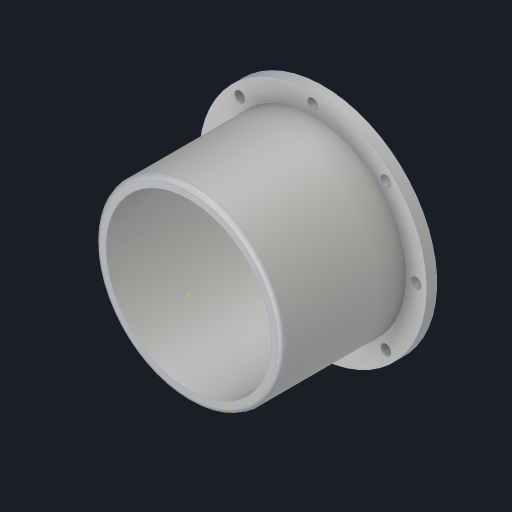
# Autodesk Inventor part: base
Saved by Autodesk Inventor 2023.4 (Build 274418000, 418)
## iProperties
Created: 2020-06-03
Part Number: base
Material: Aluminum 6061
Document SubType Name: Modeling
Designer: lenovo
Density: 2.7 g/cm^3
Appearance: Aluminum - Flat
Author: lenovo
Autodesk Inventor part; units mm, degrees
ref_plane "YZ Plane" through (0, 0, 0) normal (1, 0, 0) x (0, 1, 0)
ref_plane "XZ Plane" through (0, 0, 0) normal (0, 1, 0) x (-1, 0, 0)
ref_plane "XY Plane" through (0, 0, 0) normal (0, 0, 1) x (1, 0, 0)
sketch "Sketch1" plane through (0, 0, 0) normal (0, 0, 1) x (1, 0, 0)
  circle A0 centre (0, 0) radius 40
  circle A1 centre (0, 0) radius 45
  dimension "d0" = 80
  dimension "d1" = 5
  constraints: 2 centre point, 1 coincident
  measures "d0" diameter of A0
  measures "d1" radial gap between concentric circles of A0 A1
extrude "Extrusion1" add sketch "Sketch1" along normal blind 60
fillet "Fillet1" radius 2 1 edges at (-45, 0, 60)
sketch "Sketch2" plane through (0, 0, 0) normal (0, 0, -1) x (-1, 0, 0)
  circle A0 centre (0, 0) radius 45 projected
  circle A1 centre (0, 0) radius 55
  dimension "d5" = 10
  constraints: 1 centre point
  measures "d5" radial gap between concentric circles of A0 A1
extrude "Extrusion2" add sketch "Sketch2" along normal blind 5
sketch "Sketch3" plane through (0, 0, 0) normal (0, 0, 1) x (1, 0, 0)
  circle A0 centre (0, -49.9533) radius 2.5
  circle A1 centre (0, 0) radius 45 projected
  circle A2 centre (49.9533, 0) radius 2.5
  circle A3 centre (0, 49.9533) radius 2.5
  circle A4 centre (-49.9533, 0) radius 2.5
  dimension "d8" = 5
  dimension "d11" = 360
  constraints: 4 centre point, 9 other
  measures "d8" diameter of A0
extrude "Extrusion3" cut sketch "Sketch3" against normal through all contours A0 | A2 | A3 | A4
sketch "Sketch4" plane through (0, 0, 0) normal (0, 0, 1) x (1, 0, 0)
  line L0 (0, 0) -> (49.953, 0) construction
  circle A0 centre (35.3221, 35.3221) radius 2.5
  circle A1 centre (35.3221, -35.3221) radius 2.5
  circle A2 centre (-35.3221, -35.3221) radius 2.5
  circle A3 centre (-35.3221, 35.3221) radius 2.5
  dimension "d20" = 360
  constraints: 4 centre point, 2 coincident, 2 end point, 1 horizontal, 11 other
extrude "Extrusion4" cut sketch "Sketch4" against normal through all
sketch "Sketch5" plane through (0, 0, 60) normal (0, 0, 1) x (1, 0, 0)
  point P0 (0, 0)
body "Solid1"
